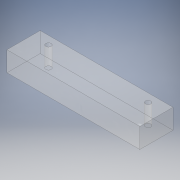
# Autodesk Inventor part: phone_holder_slider_insert
Saved by Autodesk Inventor 2019 (Build 230136000, 136)
## iProperties
Created: 2019-02-17
Part Number: phone_holder_slider_insert
Material: Acrylic, Clear
Document SubType Name: Modeling
Designer: suchanek
Density: 1.19 g/cm^3
Appearance: Transparent - Clear
Author: suchanek
Autodesk Inventor part; units mm, degrees
ref_plane "YZ Plane" through (0, 0, 0) normal (1, 0, 0) x (0, 1, 0)
ref_plane "XZ Plane" through (0, 0, 0) normal (0, 1, 0) x (-1, 0, 0)
ref_plane "XY Plane" through (0, 0, 0) normal (0, 0, 1) x (1, 0, 0)
sketch "Sketch1" plane through (0, 0, 0) normal (0, 1, 0) x (-1, 0, 0)
  line L0 (-6.308, 9.234) -> (33.692, 9.234)
  line L1 (33.692, 9.234) -> (33.692, -0.766)
  line L2 (33.692, -0.766) -> (-6.308, -0.766)
  line L3 (-6.308, -0.766) -> (-6.308, 9.234)
  circle A0 centre (-1.308, 1.734) radius 0.8
  circle A1 centre (28.692, 1.734) radius 0.8
  point P0 (0, 0)
  dimension "d0" = 1.6
  dimension "d1" = 2.5
  dimension "d2" = 5
  dimension "d3" = 5
  dimension "d4" = 30
  dimension "d5" = 10
  constraints: 8 end point, 2 centre point, 2 parallel, 1 equal radius, 1 horizontal, 1 horizontal alignment, 1 perpendicular
  measures "d0" diameter of A1
  measures "d1" distance from line of L2 A1.centre
  measures "d2" distance from line of L1 A1.centre
  measures "d3" distance from line of L3 A0.centre
  measures "d4" distance of A0.centre A1.centre
  measures "d5" distance of L0.end L1.end
extrude "Extrusion1" add sketch "Sketch1" along normal blind 6
body "Solid1"
